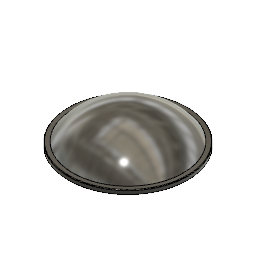
CSR_RadarEye_Lens (Autodesk Fusion 360 design; units mm, degrees)
Autodesk Fusion 360 part; units mm, degrees
sketch "Sketch1" plane through (0, 0, 0) normal (0, 0, 1) x (1, 0, 0)
  arc A0 (0, 47.625) -> (-38.1, 28.575) centre (0, 0) ccw
  line L0 (-41.275, 28.575) -> (-41.275, 25.4)
  line L1 (-41.275, 28.575) -> (-38.1, 28.575)
  line L2 (-41.275, 25.4) -> (-36.478, 25.4)
  line L3 (0, 47.625) -> (0, 44.45)
  arc A1 (0, 44.45) -> (-36.478, 25.4) centre (0, 0) ccw
  dimension "d3" = 3.175
revolve "Revolve1" add sketch "Sketch1" angle 360 about axis through (0, 47.625, 0) along (0, -1, 0)
fillet "Fillet1" radius 0.381 3 edges at (-38.4818, 25.4, 14.9257) (-38.4818, 28.575, 14.9257) (-34.0094, 25.4, 13.191)
